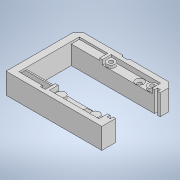
# Autodesk Inventor part: Стойка под электроннику
Saved by Autodesk Inventor 2020 (Build 240168000, 168)
## iProperties
Created: 2021-04-05
Part Number: Стойка под электроннику
Material: Типовые
Document SubType Name: Обычные детали
Designer: Антон
Density: 1 g/cm^3
Appearance: По умолчанию
Sheet Metal Rule: По умолчанию
Author: Антон
Autodesk Inventor part; units mm, degrees
ref_plane "YZ Plane" through (0, 0, 0) normal (1, 0, 0) x (0, 1, 0)
ref_plane "XZ Plane" through (0, 0, 0) normal (0, 1, 0) x (-1, 0, 0)
ref_plane "XY Plane" through (0, 0, 0) normal (0, 0, 1) x (1, 0, 0)
sketch "Эскиз1" plane through (0, 0, 0) normal (0, 1, 0) x (-1, 0, 0)
  line L0 (0, 0) -> (69, 0)
  line L1 (69, 0) -> (69, -52)
  line L2 (69, -52) -> (0, -52)
  line L3 (0, -52) -> (0, 0)
  line L4 (0, -26) -> (32, -26)
  line L5 (64, -10) -> (0, -10)
  line L6 (0, -10) -> (0, -42)
  line L7 (0, -42) -> (64, -42)
  line L8 (64, -42) -> (64, -10)
  line L9 (64, -10) -> (0, -42) construction
  line L10 (0, -10) -> (64, -42) construction
  line L11 (0, -10) -> (2, -10)
  point P0 (0, -10)
  dimension "d0" = 69
  dimension "d224" = 10
  dimension "d225" = 5
  dimension "d226" = 32
  constraints: 24 end point, 4 horizontal, 4 parallel, 3 midpoint, 2 perpendicular, 1 point on line
  measures "d0" distance of L1.end L2.end
  measures "d224" distance between parallel lines of L0 L5
  measures "d225" distance between parallel lines of L1 L8
  measures "d226" distance between parallel lines of L7 L5
extrude "Выдавливание1" add sketch "Эскиз1" along normal blind 15 contours L0 L1 L2 L3 L7 L8 L5
sketch "Эскиз2" plane through (0, 15, 0) normal (0, 1, 0) x (1, 0, 0)
  line L0 (-5.8, 3.775) -> (-41.5, 3.775)
  line L1 (-41.5, 3.775) -> (-41.5, 48.225)
  line L2 (-41.5, 48.225) -> (-5.8, 48.225)
  line L3 (-5.8, 48.225) -> (-5.8, 3.775)
  line L4 (-5.8, 3.775) -> (-41.5, 48.225) construction
  line L5 (-41.5, 3.775) -> (-5.8, 48.225) construction
  line L6 (0, 0) -> (0, 10) projected
  line L7 (-69, 52) -> (-69, 0) projected
  line L8 (-64, 4.225) -> (-43.5, 4.225)
  line L9 (-43.5, 4.225) -> (-43.5, 47.775)
  line L10 (-43.5, 47.775) -> (-64, 47.775)
  line L11 (-64, 47.775) -> (-64, 4.225)
  line L12 (0, 52) -> (-69, 52) construction
  line L13 (-64, 10) -> (-64, 42) projected
  point P0 (-23.65, 26)
  point P1 (-23.65, 26)
  point P2 (-69, 26)
  point P3 (-23.65, 26)
  point P4 (-69, 26)
  point P5 (-43.5, 26)
  point P6 (-41.5, 26)
  dimension "d227" = 35.7
  dimension "d228" = 44.45
  dimension "d233" = 20.5
  dimension "d234" = 43.55
  dimension "d235" = 2
  constraints: 20 end point, 8 midpoint, 4 parallel, 2 horizontal, 2 horizontal alignment, 2 perpendicular, 1 collinear
  measures "d227" distance of L1.end L2.end
  measures "d228" distance of L0.end L1.end
  measures "d233" distance of L9.end L10.end
  measures "d234" distance of L10.end L8.start
  measures "d235" distance between parallel lines of L9 L1
extrude "Выдавливание2" cut sketch "Эскиз2" against normal blind 3.5
sketch "Эскиз3" plane through (0, 11.5, 0) normal (0, 1, 0) x (1, 0, 0)
  circle A0 centre (-38.5, 45.225) radius 3
  circle A1 centre (-8.8, 45.225) radius 3
  line L0 (-41.5, 48.225) -> (-5.8, 48.225) projected
  line L1 (-5.8, 48.225) -> (-5.8, 42) projected
  line L2 (-5.8, 42) -> (-41.5, 42) projected
  line L3 (-41.5, 42) -> (-41.5, 48.225) projected
  circle A2 centre (-36, 6.775) radius 3
  circle A3 centre (-11.3, 6.775) radius 3
  line L4 (-5.8, 10) -> (-5.8, 3.775) projected
  line L5 (-5.8, 3.775) -> (-41.5, 3.775) projected
  line L6 (-41.5, 3.775) -> (-41.5, 10) projected
  line L7 (-64, 10) -> (-43.5, 10) projected
  line L8 (-64, 4.225) -> (-64, 10) projected
  line L9 (-43.5, 4.225) -> (-64, 4.225) projected
  line L10 (-43.5, 10) -> (-43.5, 4.225) projected
  line L11 (-43.5, 42) -> (-64, 42) projected
  line L12 (-43.5, 47.775) -> (-43.5, 42) projected
  line L13 (-64, 47.775) -> (-43.5, 47.775) projected
  line L14 (-64, 42) -> (-64, 47.775) projected
  point P0 (-38, 39.1)
  point P1 (-41.5, 45.225)
  point P2 (-8.3, 39.1)
  point P3 (-5.8, 45.225)
  point P4 (-38.5, 48.225)
  point P5 (-8.8, 48.225)
  point P6 (-5.3, 5.3)
  point P7 (-11.3, 3.775)
  point P8 (-41, 5.3)
  point P9 (-36, 3.775)
  dimension "d236" = 3
  dimension "d237" = 3
  dimension "d238" = 3
  dimension "d239" = 3
  dimension "d240" = 6
  dimension "d241" = 6
  dimension "d242" = 5.5
  dimension "d244" = 3
  dimension "d245" = 6
  dimension "d246" = 5.5
  dimension "d247" = 3
  dimension "d248" = 6
  constraints: 4 centre point
  measures "d236" distance from line of L0 A1.centre
  measures "d237" distance from line of L1 A1.centre
  measures "d238" distance from line of L3 A0.centre
  measures "d239" distance from line of L0 A0.centre
  measures "d240" diameter of A0
  measures "d241" diameter of A1
  measures "d242" distance from line of L4 A3.centre
  measures "d244" distance from line of L5 A3.centre
  measures "d245" diameter of A3
  measures "d246" distance from line of L6 A2.centre
  measures "d247" distance from line of L5 A2.centre
  measures "d248" diameter of A2
extrude "Выдавливание5" add sketch "Эскиз3" along normal blind 2 contours A0 | A0 L3 L0 | L0 L1 A1 | A1 | A2 | A3 | L7 L10 L9 L8 | L11 L14 L13 L12
sketch "Эскиз4" plane through (-71.3, 13.5, -19.65) normal (0, 1, 0) x (0, 0, -1)
  arc A0 (25.575, -29.8) -> (28.575, -32.8) centre (25.575, -32.8) ccw projected
  arc A1 (28.575, -62.5) -> (25.575, -65.5) centre (25.575, -62.5) ccw projected
hole "Отверстие1" at (-38.5, 13.5, -45.225) at (-8.8, 13.5, -45.225) direction (0, -1, 0) diameter 3 depth 5
sketch "Эскиз32" plane through (0, 11.5, 0) normal (0, 1, 0) x (1, 0, 0)
  line L0 (-64, 4.225) -> (-64, 47.775) projected
  line L1 (-64, 47.775) -> (-43.5, 47.775) projected
  line L2 (-5.8, 3.775) -> (-41.5, 3.775) projected
  circle A0 centre (-11.3, 6.775) radius 3 projected
  line L3 (-5.8, 10) -> (-5.8, 3.775) projected
  line L4 (-41.5, 48.225) -> (-5.8, 48.225) projected
  line L5 (-5.8, 48.225) -> (-5.8, 42) projected
  point P0 (0, 0)
  point P1 (-17.8, 6.8875)
  point P2 (-5.3, 5.3)
  point P3 (-8.3, 2.3)
  point P4 (-17.8, 45.1125)
  dimension "d261" = 3.1125
  dimension "d263" = 12
  dimension "d296" = 3.1125
  dimension "d297" = 12
  constraints: 3 other
  measures "d296" distance from line of L4 point (-17.8, 45.112)
  measures "d297" distance from line of L5 point (-17.8, 45.112)
hole "Отверстие5" at (-17.8, 11.5, -6.8875) at (-17.8, 11.5, -45.1125) direction (0, -1, 0) diameter 3.2 end through all countersink diameter 6 countersink angle 90
sketch "Эскиз12" plane through (0, 15, 0) normal (0, -1, 0) x (1, 0, 0)
  line L0 (-41.5, -48.225) -> (-5.8, -48.225) projected
  line L1 (0, -52) -> (-69, -52) projected
  line L2 (-35.9, -52) -> (-33.1, -52) construction
  line L3 (-35.9, -53) -> (-33.1, -53)
  line L4 (-33.1, -51) -> (-35.9, -51)
  arc A0 (-35.9, -51) -> (-35.9, -53) centre (-35.9, -52) ccw
  arc A1 (-33.1, -53) -> (-33.1, -51) centre (-33.1, -52) ccw
  point P0 (-34.5, -52)
  dimension "d302" = 1.4
  dimension "d303" = 2
  constraints: 8 end point, 4 point on circle, 4 tangent, 2 centre point, 2 midpoint, 1 parallel, 1 point on line
  measures "d302" distance of point (-34.5, -52) L2.end
  measures "d303" diameter of A1
extrude "Выдавливание11" cut sketch "Эскиз12" along normal through all
sketch "Эскиз34" plane through (0, 15, 0) normal (0, 1, 0) x (1, 0, 0)
  line L0 (-4, 7.9) -> (-1.8, 7.9)
  line L1 (-1.8, 7.9) -> (-1.8, 10)
  line L2 (-1.8, 10) -> (-4, 10)
  line L3 (-4, 10) -> (-4, 7.9)
  line L4 (0, 10) -> (-5.8, 10) projected
  line L5 (-4, 42) -> (-1.8, 42)
  line L6 (-1.8, 42) -> (-1.8, 44.1)
  line L7 (-1.8, 44.1) -> (-4, 44.1)
  line L8 (-4, 44.1) -> (-4, 42)
  line L9 (-5.8, 42) -> (0, 42) projected
  point P0 (0, 0)
  point P1 (-2.9, 10)
  point P2 (-2.9, 42)
  dimension "d278" = 2.2
  dimension "d279" = 2.1
  constraints: 16 end point, 4 midpoint, 4 parallel, 2 equal length, 2 horizontal, 2 perpendicular
  measures "d278" distance between parallel lines of L1 L3
  measures "d279" distance of L2.end L0.start
extrude "Выдавливание27" cut sketch "Эскиз34" against normal through all
sketch "Эскиз36" plane through (0, 0, 0) normal (0, -1, 0) x (1, 0, 0)
  line L0 (-64, -10) -> (-64, 0)
  line L1 (-69, 0) -> (0, 0) projected
  line L2 (-67, -9) -> (-42, -9)
  line L3 (-42, -9) -> (-42, -1)
  line L4 (-42, -1) -> (-67, -1)
  line L5 (-67, -1) -> (-67, -9)
  line L6 (-69, -52) -> (-69, 0) projected
  point P0 (-67, -5)
  point P1 (-64, -5)
  dimension "d285" = 2
  dimension "d286" = 8
  dimension "d287" = 25
  constraints: 10 end point, 2 midpoint, 2 parallel, 1 coincident, 1 horizontal, 1 horizontal alignment, 1 perpendicular, 1 point on line, 1 vertical
  measures "d285" distance between parallel lines of L6 L5
  measures "d286" distance of L2.end L3.end
  measures "d287" distance of L3.end L4.end
extrude "Выдавливание29" cut sketch "Эскиз36" against normal blind 13.5
sketch "Эскиз37" plane through (-69, 0, -52) normal (-1, 0, 0) x (0, 0, 1)
  line L0 (43, 0) -> (51, 0) projected
  line L1 (43, 0) -> (43, 13.5) projected
  line L2 (43, 13.5) -> (51, 13.5) projected
  line L3 (51, 0) -> (51, 13.5) projected
  line L4 (43, 0) -> (43, 13.5) construction
  line L5 (43, 6.75) -> (51, 6.75) construction
  line L6 (51, 0) -> (51, 13.5) construction
  circle A0 centre (47, 6.75) radius 3.25
  point P0 (52, 0)
  dimension "d290" = 6.5
  constraints: 3 midpoint, 2 end point, 1 centre point
  measures "d290" diameter of A0
extrude "Выдавливание30" cut sketch "Эскиз37" against normal up to surface (2 mm away) contours A0
sketch "Эскиз38" plane through (0, 15, 0) normal (0, 1, 0) x (1, 0, 0)
  line L0 (-43.5, 10) -> (-43.5, 4.225) projected
  line L1 (-43.5, 4.225) -> (-47, 4.225)
  line L2 (-47, 4.225) -> (-47, 2.725)
  line L3 (-47, 2.725) -> (-43.5, 2.725)
  line L4 (-43.5, 2.725) -> (-43.5, 4.225)
  line L5 (-69, 0) -> (0, 0) projected
  dimension "d293" = 3.5
  dimension "d301" = 1.5
  constraints: 8 end point, 2 parallel, 1 horizontal, 1 perpendicular
  measures "d293" distance of L3.end L2.end
  measures "d301" distance of L1.end L2.end
extrude "Выдавливание31" cut sketch "Эскиз38" against normal up to surface (1.5 mm away)
sketch "Эскиз30" plane through (0, 0, 0) normal (0, -1, 0) x (1, 0, 0)
  line L0 (-69, -39.85) -> (-67, -39.85)
  line L1 (-67, -39.85) -> (-67, -12.15)
  line L2 (-67, -12.15) -> (-69, -12.15)
  line L3 (-69, -12.15) -> (-69, -39.85)
  line L4 (-69, -52) -> (-69, 0) projected
  line L5 (-67, -39.85) -> (-68.1, -39.85)
  line L6 (-68.1, -39.85) -> (-68.1, -40.85)
  line L7 (-68.1, -40.85) -> (-67, -40.85)
  line L8 (-67, -40.85) -> (-67, -39.85)
  line L9 (-67, -12.15) -> (-68.5, -12.15)
  line L10 (-68.5, -12.15) -> (-68.5, -11.15)
  line L11 (-68.5, -11.15) -> (-67, -11.15)
  line L12 (-67, -11.15) -> (-67, -12.15)
  point P0 (0, 0)
  point P1 (-69, -26)
  point P2 (-68.5, -12.15)
  point P3 (-68.1, -39.85)
  dimension "d216" = 27.7
  dimension "d217" = 2
  dimension "d218" = 1.1
  dimension "d219" = 1
  dimension "d220" = 1.5
  dimension "d221" = 1
  constraints: 24 end point, 6 parallel, 3 horizontal, 3 perpendicular, 2 midpoint
  measures "d216" distance of L0.end L1.end
  measures "d217" distance of L0.start L0.end
  measures "d218" distance of L7.end L6.end
  measures "d219" distance of L7.end L0.end
  measures "d220" distance of L10.end L11.end
  measures "d221" distance of L9.end L10.end
extrude "Выдавливание24" cut sketch "Эскиз30" against normal blind 13.1
chamfer "Фаска7" distance 4 angle 45 2 edges at (0, 7.5, -52) (-69, 7.5, -52)
